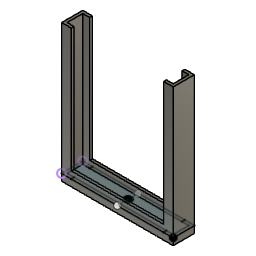
pan holder 2 v4 (Autodesk Fusion 360 design; units mm, degrees)
Autodesk Fusion 360 part; units mm, degrees
sketch "Sketch1" plane through (0, 0, 0) normal (0, 0, 1) x (1, 0, 0)
  line L0 (0, 0) -> (81.3, 0)
  line L1 (81.3, 0) -> (81.3, 15.4)
  line L2 (81.3, 15.4) -> (0, 15.4)
  line L3 (0, 15.4) -> (0, 0)
  dimension "d8" = 81.3
  dimension "d9" = 15.4
  constraint horizontal L0
  constraint vertical L1
  constraint horizontal L2
  constraint vertical L3
  constraint coincident L0.start L3.end
  measures "d8" distance of L0.start L0.end
  measures "d9" distance of L0.start L2.end
extrude "Extrude1" add sketch "Sketch1" along normal blind 5
sketch "Sketch2" plane through (0, 0, 5) normal (0, 0, 1) x (-1, 0, 0)
  line L0 (0, -15.4) -> (0, 0)
  line L1 (0, 0) -> (-81.3, 0)
  line L2 (-81.3, 0) -> (-81.3, -15.4)
  line L3 (-81.3, -15.4) -> (0, -15.4)
  circle A0 centre (-40.65, -7.7) radius 1.65
  circle A1 centre (-40.65, -7.7) radius 2.725
  dimension "d16" = 3.3
  dimension "d17" = 40.65
  dimension "d18" = 7.7
  dimension "d19" = 5.45
  constraint concentric A0 A1
  measures "d16" diameter of A0
  measures "d17" distance of L0 A0.centre
  measures "d18" distance of L3 A0.centre
  measures "d19" diameter of A1
extrude "Extrude2" cut sketch "Sketch2" against normal blind 5 contours A0
extrude "Extrude3" cut sketch "Sketch2" against normal blind 3.1 contours A1
sketch "Sketch3" plane through (0, 0, 5) normal (0, 0, 1) x (1, 0, 0)
  line L0 (40.65, 14.9854) -> (40.65, -0.0146) construction
  line L1 (0, 15.4) -> (0, 0) construction
  line L2 (74.3, 15.4) -> (74.3, 13.4)
  line L3 (74.3, 13.4) -> (79.3, 13.4)
  line L4 (79.3, 13.4) -> (79.3, 2)
  line L5 (79.3, 2) -> (74.3, 2)
  line L6 (74.3, 2) -> (74.3, 0)
  line L7 (74.3, 0) -> (81.3, 0)
  line L8 (81.3, 0) -> (81.3, 15.4)
  line L9 (81.3, 15.4) -> (74.3, 15.4)
  line L10 (0, 0) -> (0, 15.4)
  line L11 (2, 13.4) -> (2, 2)
  line L12 (2, 2) -> (7, 2)
  line L13 (7, 13.4) -> (2, 13.4)
  line L14 (7, 0) -> (0, 0)
  line L15 (7, 15.4) -> (7, 13.4)
  line L16 (0, 15.4) -> (7, 15.4)
  line L17 (7, 2) -> (7, 0)
  line L18 (7, 15.4) -> (74.3, 15.4)
  line L19 (74.3, 15.4) -> (74.3, 13.4)
  line L20 (74.3, 13.4) -> (7, 13.4)
  line L21 (7, 13.4) -> (7, 15.4)
  line L22 (74.3, 2) -> (7, 2)
  line L23 (7, 2) -> (7, 0)
  line L24 (7, 0) -> (74.3, 0)
  line L25 (74.3, 0) -> (74.3, 2)
  point P0 (81.3, 0)
  dimension "d24" = 40.65
  dimension "d25" = 2
  dimension "d26" = 15.4
  dimension "d27" = 2
  dimension "d29" = 5
  constraint vertical L0
  constraint vertical L2
  constraint perpendicular L2 L3
  constraint perpendicular L3 L4
  constraint perpendicular L2 L5
  constraint perpendicular L5 L6
  constraint perpendicular L6 L7
  constraint perpendicular L5 L8
  constraint perpendicular L2 L9
  constraint equal L2 L6
  constraint equal L3 L5
  constraint symmetric L0 L2.start L15.start
  constraint symmetric L0 L2.end L13.start
  constraint symmetric L0 L3.end L11.start
  constraint symmetric L0 L4.end L11.end
  constraint symmetric L0 L5.end L12.end
  constraint symmetric L0 L6.end L14.start
  constraint symmetric L0 P0 L1.end
  constraint symmetric L0 L8.end L1.start
  constraint coincident P0 L7.end
  constraint horizontal L18
  constraint vertical L19
  constraint horizontal L20
  constraint vertical L21
  constraint horizontal L22
  constraint vertical L23
  constraint horizontal L24
  constraint vertical L25
  measures "d24" distance of L0 L1
  measures "d25" distance of L2.start L2.end
  measures "d26" distance of P0 L8.end
  measures "d27" distance of L4 L8
  measures "d29" distance of L2.end L3.end
extrude "Extrude4" add sketch "Sketch3" along normal blind 95.16 contours L2 L3 L4 L5 L6 L7 L8 L9 L19 L25 | L10 L11 L12 L13 L14 L15 L16 L17 L21 L23
extrude "Extrude5" add sketch "Sketch3" along normal blind 5 contours L2 L15 L18 L19 L20 L21 | L6 L17 L22 L23 L24 L25
equation "pw = 74.8 mm"
equation "pd = 8.9 mm"
equation "ph = 158.6 mm"
equation "clearance = 1.25 mm"
equation "wall_thick = 2 mm"
equation "outer_w = 2 * clearance + 2 * wall_thick + pw"
equation "outer_d = 2 * clearance + 2 * wall_thick + pd"
equation "d8 = outer_w"
equation "d9 = outer_d"
equation "d17 = outer_w / 2"
equation "d18 = outer_d / 2"
equation "d24 = outer_w / 2"
equation "d25 = wall_thick"
equation "d26 = outer_d"
equation "d27 = wall_thick"
equation "d30 = ph * 0.6"
